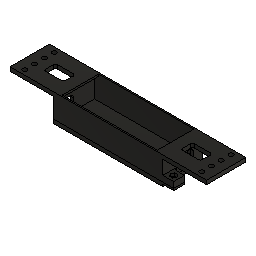
ports_usb_hub (Autodesk Fusion 360 design; units mm, degrees)
Autodesk Fusion 360 part; units mm, degrees
sketch "Sketch1" plane through (0, 0, 0) normal (0, 0, 1) x (1, 0, 0)
  line L0 (0, 0) -> (105, 0)
  line L1 (105, 0) -> (105, -36)
  line L2 (105, -36) -> (0, -36)
  line L3 (0, -36) -> (0, 0)
  line L4 (0, 0) -> (105, -36) construction
  line L5 (105, 0) -> (100, 0) construction
  line L6 (0, -36) -> (105, 0) construction
  line L7 (132.5, 2) -> (-27.5, 2)
  line L8 (-27.5, 2) -> (-27.5, -38)
  line L9 (-27.5, -38) -> (132.5, -38)
  line L10 (132.5, -38) -> (132.5, 2)
  line L11 (132.5, 2) -> (-27.5, -38) construction
  line L12 (-27.5, 2) -> (132.5, -38) construction
  line L13 (-27.5, 2) -> (-47.5, 2)
  line L14 (-47.5, 2) -> (-47.5, -38)
  line L15 (-47.5, -38) -> (-27.5, -38)
  line L16 (-27.5, -38) -> (-27.5, 2)
  line L17 (132.5, 2) -> (152.5, 2)
  line L18 (152.5, 2) -> (152.5, -38)
  line L19 (152.5, -38) -> (132.5, -38)
  line L20 (132.5, -38) -> (132.5, 2)
  line L21 (-37.5, 2) -> (-37.5, -38) construction
  line L22 (142.5, 2) -> (142.5, -38) construction
  line L23 (142.5, 2) -> (142.5, -3) construction
  line L24 (-37.5, 2) -> (-37.5, -3) construction
  circle A0 centre (142.5, -3) radius 2.2
  circle A1 centre (-37.5, -3) radius 2.2
  circle A2 centre (-37.5, -13) radius 2.2
  circle A3 centre (142.5, -13) radius 2.2
  circle A4 centre (-37.5, -23) radius 2.2
  circle A5 centre (142.5, -23) radius 2.2
  circle A6 centre (-37.5, -33) radius 2.2
  circle A7 centre (142.5, -33) radius 2.2
  line L25 (-3, 2) -> (108, 2)
  line L26 (108, 2) -> (108, -38)
  line L27 (108, -38) -> (-3, -38)
  line L28 (-3, -38) -> (-3, 2)
  line L29 (-3, 2) -> (108, -38) construction
  line L30 (108, 2) -> (-3, -38) construction
  point P0 (52.5, -18)
  point P1 (52.5, -18)
  dimension "d1" = 105
  dimension "d2" = 36
  dimension "d3" = 160
  dimension "d4" = 40
  dimension "d5" = 40
  dimension "d6" = 20
  dimension "d7" = 40
  dimension "d8" = 20
  dimension "d9" = 5
  dimension "d10" = 5
  dimension "d11" = 4.4
  dimension "d12" = 4.4
  dimension "d15" = 10
  dimension "d16" = -10
  dimension "d17" = 111
  dimension "d18" = 40
  constraint horizontal L0
  constraint vertical L1
  constraint horizontal L2
  constraint vertical L3
  constraint coincident L0.start L3.end
  constraint coincident L0 L5.end
  constraint perpendicular L7 L8
  constraint parallel L7 L9
  constraint parallel L8 L10
  constraint horizontal L7
  constraint coincident L11 P1
  constraint coincident L12 P1
  constraint midpoint L4 P1
  constraint horizontal L13
  constraint vertical L14
  constraint horizontal L15
  constraint vertical L16
  constraint horizontal L17
  constraint vertical L18
  constraint horizontal L19
  constraint vertical L20
  constraint midpoint L13 L21.start
  constraint midpoint L15 L21.end
  constraint midpoint L17 L22.start
  constraint midpoint L19 L22.end
  constraint perpendicular L17 L23
  constraint perpendicular L13 L24
  constraint coincident L23.end A0.centre
  constraint coincident L24.end A1.centre
  constraint perpendicular L25 L26
  constraint parallel L25 L27
  constraint parallel L26 L28
  constraint horizontal L25
  constraint coincident L29 P1
  constraint coincident L30 P1
  constraint coincident P1 P0
  measures "d1" distance of L0.start L0.end
  measures "d2" distance of L0.start L2.end
  measures "d3" distance of L8.end L9.end
  measures "d4" distance of L7.end L8.end
  measures "d5" distance of L7.end L8.end
  measures "d6" distance of L7.end L13.end
  measures "d7" distance of L7.start L9.end
  measures "d8" distance of L7.start L17.end
  measures "d9" distance of L22.start L23.end
  measures "d10" distance of L21.start L24.end
  measures "d11" diameter of A0
  measures "d12" diameter of A1
  measures "d17" distance of L26.end L27.end
  measures "d18" distance of L25.end L26.end
extrude "Extrude1" add sketch "Sketch1" along normal blind 4 makes body 1
extrude "Extrude2" add sketch "Sketch1" against normal blind 20 contours L7 L9 L25 L26 L27 L28 bodies 1
sketch "Sketch2" plane through (0, 0, -20) normal (0, 0, -1) x (1, 0, 0)
  line L0 (0, 36) -> (105, 36)
  line L1 (105, 36) -> (105, 0)
  line L2 (105, 0) -> (0, 0)
  line L3 (0, 0) -> (0, 36)
  line L4 (108, 38) -> (-3, 38)
  line L5 (-3, 38) -> (-3, -2)
  line L6 (-3, -2) -> (108, -2)
  line L7 (108, -2) -> (108, 38)
  line L8 (108, -2) -> (108, 7) construction
  line L9 (108, 7) -> (105, 7)
  line L10 (105, 7) -> (105, 15)
  line L11 (105, 15) -> (108, 15)
  line L12 (108, 15) -> (108, 7)
  line L13 (-3, 38) -> (-3, 29) construction
  line L14 (-3, 29) -> (0, 29)
  line L15 (0, 29) -> (0, 21)
  line L16 (0, 21) -> (-3, 21)
  line L17 (-3, 21) -> (-3, 29)
  dimension "d23" = 9
  dimension "d24" = 8
  dimension "d25" = 9
  dimension "d26" = 8
  constraint coincident L6.end L7.start
  constraint perpendicular L6 L8
  constraint horizontal L9
  constraint vertical L10
  constraint horizontal L11
  constraint vertical L12
  constraint coincident L4.end L5.start
  constraint perpendicular L4 L13
  constraint horizontal L14
  constraint vertical L15
  constraint horizontal L16
  constraint vertical L17
  measures "d23" distance of L6.end L8.end
  measures "d24" distance of L8.end L11.end
  measures "d25" distance of L4.end L13.end
  measures "d26" distance of L13.end L16.end
extrude "Extrude3" cut sketch "Sketch2" against normal blind 15 contours L3 L5 L14 L15 L16 L17 | L1 L7 L9 L10 L11 L12 bodies 1
fillet "Fillet1" radius 3 2 edges at (-1.5, -21, -5) (-1.5, -29, -5) on bodies 1
fillet "Fillet1" radius 3 2 edges at (106.5, -7, -5) (106.5, -15, -5) on bodies 1
sketch "Sketch3" plane through (0, 0, 4) normal (0, 0, 1) x (-1, 0, 0)
  circle A0 centre (-142.5, 33) radius 2.2
  circle A1 centre (37.5, 33) radius 2.2
  circle A2 centre (-142.5, 13) radius 2.2
  circle A3 centre (37.5, 23) radius 2.2
  circle A4 centre (-142.5, 23) radius 2.2
  circle A5 centre (37.5, 13) radius 2.2
  circle A6 centre (37.5, 3) radius 2.2
  circle A7 centre (-142.5, 3) radius 2.2
  line L0 (-105, 36) -> (0, 36)
  line L1 (0, 36) -> (0, 0)
  line L2 (0, 0) -> (-105, 0)
  line L3 (-105, 0) -> (-105, 36)
  line L4 (-152.5, -2) -> (47.5, -2)
  line L5 (47.5, -2) -> (47.5, 38)
  line L6 (47.5, 38) -> (-152.5, 38)
  line L7 (-152.5, 38) -> (-152.5, -2)
  line L8 (-52.5, 0) -> (-52.5, 36) construction
  line L9 (0, 0) -> (-3, 0)
  line L10 (-3, 0) -> (-3, 36)
  line L11 (-3, 36) -> (0, 36)
  line L12 (0, 36) -> (0, 0)
  line L13 (-102, 0) -> (-102, 36)
  dimension "d30" = 3
  constraint midpoint L2 L8.start
  constraint midpoint L0 L8.end
  constraint horizontal L9
  constraint vertical L10
  constraint horizontal L11
  constraint vertical L12
  constraint coincident L1.end L2.start
  constraint symmetric L8 L9.end L13.start
  constraint symmetric L8 L10.end L13.end
  measures "d30" distance of L1.end L9.end
extrude "Extrude4" add sketch "Sketch3" against normal blind 2 contours L0 L2 L3 L13 | L0 L1 L2 L9 L10 L11 L12 bodies 1
sketch "Sketch4" plane through (0, 0, -20) normal (0, 0, -1) x (1, 0, 0)
  line L0 (105, 7) -> (105, 0)
  line L1 (105, 0) -> (0, 0)
  line L2 (0, 0) -> (0, 21)
  line L3 (-3, 21) -> (-3, -2)
  line L4 (-3, -2) -> (108, -2)
  line L5 (108, -2) -> (108, 7)
  line L6 (0, 21) -> (-11, 21)
  line L7 (-11, 21) -> (-11, 10)
  line L8 (-11, 10) -> (0, 10)
  line L9 (0, 10) -> (0, 21)
  line L10 (0, 21) -> (-11, 10) construction
  circle A0 centre (-5.5, 15.5) radius 1.75
  line L11 (108, 7) -> (105, 7)
  line L12 (0, 21) -> (-3, 21)
  dimension "d33" = 11
  dimension "d34" = 11
  dimension "d35" = 3.5
  constraint horizontal L6
  constraint vertical L7
  constraint horizontal L8
  constraint vertical L9
  constraint coincident L2.end L6.start
  constraint midpoint L10 A0.centre
  measures "d33" distance of L2.end L6.end
  measures "d34" distance of L2.end L8.end
  measures "d35" diameter of A0
sketch "Sketch5" plane through (0, 0, -20) normal (0, 0, -1) x (1, 0, 0)
  line L0 (108, 7) -> (105, 7)
  line L1 (105, 7) -> (105, 0)
  line L2 (105, 0) -> (0, 0)
  line L3 (0, 0) -> (0, 21)
  line L4 (0, 21) -> (-3, 21)
  line L5 (-3, 21) -> (-3, -2)
  line L6 (-3, -2) -> (108, -2)
  line L7 (108, -2) -> (108, 7)
  line L8 (-3, -2) -> (-14, -2)
  line L9 (-14, -2) -> (-14, 9)
  line L10 (-14, 9) -> (-3, 9)
  line L11 (-3, 9) -> (-3, -2)
  circle A0 centre (-8.5, 3.5) radius 1.75
  dimension "d37" = 11
  dimension "d38" = 11
  dimension "d39" = 3.5
  constraint horizontal L8
  constraint vertical L9
  constraint horizontal L10
  constraint vertical L11
  constraint coincident L5.end L6.start
  measures "d37" distance of L5.end L10.end
  measures "d38" distance of L5.end L8.end
  measures "d39" diameter of A0
extrude "Extrude5" add sketch "Sketch5" against normal blind 20 separate body contours L5 L8 L9 L10 L11 makes body 2
sketch "Sketch6" plane through (0, 2, 0) normal (0, 1, 0) x (-1, 0, 0)
  line L0 (3, -20) -> (14, -20)
  line L1 (14, -20) -> (14, 0)
  line L2 (14, 0) -> (3, 0)
  line L3 (3, 0) -> (3, -20)
  line L4 (3, -20) -> (14, -20)
  line L5 (14, -20) -> (14, -17)
  line L6 (14, -17) -> (3, -17)
  line L7 (3, -17) -> (3, -20)
  line L8 (3, -17) -> (14, -17)
  line L9 (14, -17) -> (14, -14)
  line L10 (14, -14) -> (3, -14)
  line L11 (3, -14) -> (3, -17)
  dimension "d42" = 3
  dimension "d43" = 3
  constraint horizontal L4
  constraint vertical L5
  constraint horizontal L6
  constraint vertical L7
  constraint coincident L0.start L3.end
  constraint horizontal L8
  constraint vertical L9
  constraint horizontal L10
  constraint vertical L11
  measures "d42" distance of L0.start L6.end
  measures "d43" distance of L6.end L10.end
extrude "Extrude6" cut sketch "Sketch6" against normal blind 17.5 contours L1 L2 L3 L10 bodies 2
sketch "Sketch7" plane through (0, 0, -14) normal (0, 0, 1) x (-1, 0, 0)
  line L0 (14, 9) -> (3, 9)
  line L1 (3, 9) -> (3, -2)
  line L2 (3, -2) -> (14, -2)
  line L3 (14, -2) -> (14, 9)
  circle A0 centre (8.5, 3.5) radius 1.75
  line L4 (10.1166, 0.7) -> (11.7332, 3.5)
  line L5 (11.7332, 3.5) -> (10.1166, 6.3)
  line L6 (10.1166, 6.3) -> (6.8834, 6.3)
  line L7 (6.8834, 6.3) -> (5.2668, 3.5)
  line L8 (5.2668, 3.5) -> (6.8834, 0.7)
  line L9 (6.8834, 0.7) -> (10.1166, 0.7)
  point P0 (8.5, 3.5)
  dimension "d46" = 2.8
  constraint coincident P0 A0.centre
  measures "d46" distance of P0 L9
extrude "Extrude7" cut sketch "Sketch7" against normal blind 3 contours L4 L5 L6 L7 L8 L9 bodies 2
copy_body "CopyPasteBodies1" bodies 2 makes body 3
move_body "Move1" bodies 3 to x (1, 0, 0) y (0, 1, 0) z (0, 0, 1) at (122, -29, 0)
sketch "Sketch8" plane through (0, 0, -20) normal (0, 0, -1) x (1, 0, 0)
  circle A0 centre (-8.5, 3.5) radius 1.75
  line L0 (-3, 9) -> (-14, 9)
  line L1 (-14, 9) -> (-14, -2)
  line L2 (-14, -2) -> (-3, -2)
  line L3 (-3, -2) -> (-3, 9)
  line L4 (119, 27) -> (108, 27)
  line L5 (108, 27) -> (108, 38)
  line L6 (108, 38) -> (119, 38)
  line L7 (119, 38) -> (119, 27)
  line L8 (108, 38) -> (-3, 38)
  line L9 (-3, 38) -> (-3, -2)
  line L10 (-3, -2) -> (108, -2)
  line L11 (108, -2) -> (108, 38)
  circle A1 centre (-8.5, 3.5) radius 1.75
  circle A2 centre (113.5, 32.5) radius 1.75
  dimension "d49" = 3.5
  constraint horizontal L4
  constraint vertical L5
  constraint horizontal L6
  constraint vertical L7
  constraint horizontal L8
  constraint vertical L9
  constraint horizontal L10
  constraint vertical L11
  constraint coincident L2.end L3.start
  constraint concentric A0 A1
  measures "d49" diameter of A2
extrude "Extrude8" add sketch "Sketch8" along normal blind 2 separate body makes body 4
copy_body "Body->Comp1" bodies 1 removing the originals makes body 5 in component "Hub Mount"
copy_body "Body->Comp1'" bodies 5 removing the originals makes body 6 in component "Front"
copy_body "CutPasteBodies1" bodies 2 3 removing the originals makes body 7 makes body 8 in component "Front"
copy_body "Body->Comp2" bodies 4 removing the originals makes body 9 in component "Back plate"
sketch "Sketch9" plane through (0, 0, 4) normal (0, 0, 1) x (-1, 0, 0)
  circle A0 centre (-142.5, 33) radius 2.2
  circle A1 centre (37.5, 33) radius 2.2
  circle A2 centre (-142.5, 23) radius 2.2
  circle A3 centre (37.5, 23) radius 2.2
  circle A4 centre (-142.5, 13) radius 2.2
  circle A5 centre (37.5, 13) radius 2.2
  circle A6 centre (37.5, 3) radius 2.2
  circle A7 centre (-142.5, 3) radius 2.2
  line L0 (-102, 36) -> (-3, 36)
  line L1 (-3, 36) -> (-3, 0)
  line L2 (-3, 0) -> (-102, 0)
  line L3 (-102, 0) -> (-102, 36)
  line L4 (-152.5, -2) -> (47.5, -2)
  line L5 (47.5, -2) -> (47.5, 38)
  line L6 (47.5, 38) -> (-152.5, 38)
  line L7 (-152.5, 38) -> (-152.5, -2)
  line L8 (-52.5, -2) -> (-52.5, 38) construction
  line L9 (-152.5, 18) -> (47.5, 18) construction
  line L10 (47.5, 18) -> (27.5, 18) construction
  line L11 (27.5, 18) -> (27.5, -2) construction
  line L12 (27.5, 18) -> (27.5, 38) construction
  line L13 (7, -2) -> (7, 38) construction
  line L14 (7, 38) -> (27.5, -2) construction
  line L15 (25.25, 12) -> (9.25, 12)
  line L16 (7.25, 14) -> (7.25, 22)
  line L17 (9.25, 24) -> (25.25, 24)
  line L18 (27.25, 22) -> (27.25, 14)
  line L19 (27.25, 12) -> (7.25, 24) construction
  line L20 (7.25, 12) -> (27.25, 24) construction
  arc A8 (25.25, 12) -> (27.25, 14) centre (25.25, 14) ccw
  arc A9 (7.25, 14) -> (9.25, 12) centre (9.25, 14) ccw
  arc A10 (9.25, 24) -> (7.25, 22) centre (9.25, 22) ccw
  arc A11 (27.25, 22) -> (25.25, 24) centre (25.25, 22) ccw
  arc A12 (-114.25, 12) -> (-112.25, 14) centre (-114.25, 14) ccw
  line L21 (-112.25, 14) -> (-112.25, 22)
  arc A13 (-112.25, 22) -> (-114.25, 24) centre (-114.25, 22) ccw
  line L22 (-114.25, 24) -> (-130.25, 24)
  arc A14 (-130.25, 24) -> (-132.25, 22) centre (-130.25, 22) ccw
  line L23 (-132.25, 22) -> (-132.25, 14)
  arc A15 (-132.25, 14) -> (-130.25, 12) centre (-130.25, 14) ccw
  line L24 (-130.25, 12) -> (-114.25, 12)
  point P0 (17.25, 18)
  dimension "d52" = 20
  dimension "d53" = 20
  dimension "d54" = 12
  dimension "d55" = 2
  constraint midpoint L4 L8.start
  constraint midpoint L6 L8.end
  constraint midpoint L7 L9.start
  constraint midpoint L5 L9.end
  constraint perpendicular L5 L10
  constraint coincident L4 L11.end
  constraint perpendicular L4 L11
  constraint coincident L6 L12.end
  constraint perpendicular L6 L12
  constraint coincident L4 L13.start
  constraint coincident L6 L13.end
  constraint perpendicular L6 L13
  constraint perpendicular L15 L16
  constraint parallel L15 L17
  constraint parallel L16 L18
  constraint horizontal L15
  constraint coincident L19 P0
  constraint coincident L20 P0
  constraint midpoint L14 P0
  constraint coincident L19.start L18
  constraint coincident L19.start L15
  constraint tangent L18 A8
  constraint tangent L15 A8
  constraint coincident L20.start L16
  constraint coincident L20.start L15
  constraint tangent L16 A9
  constraint tangent L15 A9
  constraint equal A8 A9
  constraint coincident L19.end L17
  constraint coincident L19.end L16
  constraint tangent L17 A10
  constraint tangent L16 A10
  constraint equal A8 A10
  constraint coincident L20.end L17
  constraint coincident L20.end L18
  constraint tangent L17 A11
  constraint tangent L18 A11
  constraint equal A8 A11
  constraint symmetric L8 L18.end L23.end
  constraint symmetric L8 L15.start A15.end
  constraint symmetric L8 A8 A15
  constraint symmetric L8 L16.start A12.end
  constraint symmetric L8 L15.end A12.start
  constraint symmetric L8 A9 A12
  constraint symmetric L8 L17.start A13.end
  constraint symmetric L8 L16.end L21.end
  constraint symmetric L8 A10 A13
  constraint symmetric L8 L17.end L22.end
  constraint symmetric L8 L18.start A14.end
  constraint symmetric L8 A11 A14
  measures "d52" distance of L9.end L10.end
  measures "d53" distance of L19.end L20.end
  measures "d54" distance of L20.start L19.end
  measures "d55" radius of A8
extrude "Extrude1'" cut sketch "Sketch9" against normal blind 20 contours L15 L16 L17 L18 A8 A9 A10 A11 | A12 L21 A13 L22 A14 L23 A15 L24 bodies 6 in component "Front"
combine "Combine1" operation add target body 6 tool bodies 8 7 in component "Front"
fillet "Fillet1'" radius 3 1 edges at (-3, -9, -21) on bodies 9 in component "Back plate"
fillet "Fillet1''" radius 3 1 edges at (108, -27, -17) on bodies 6 in component "Front"
fillet "Fillet2" radius 3 1 edges at (108, -27, -21) on bodies 9 in component "Back plate"
fillet "Fillet2'" radius 3 1 edges at (-3, -9, -17) on bodies 6 in component "Front"
sketch "Sketch10" plane through (0, 0, -22) normal (0, 0, -1) x (1, 0, 0)
  circle A0 centre (113.5, 32.5) radius 1.75
  circle A1 centre (-8.5, 3.5) radius 1.75
  line L0 (119, 38) -> (-3, 38)
  line L1 (-3, 38) -> (-3, 12)
  arc A2 (-6, 9) -> (-3, 12) centre (-6, 12) ccw
  line L2 (-6, 9) -> (-14, 9)
  line L3 (-14, 9) -> (-14, -2)
  line L4 (-14, -2) -> (108, -2)
  line L5 (108, -2) -> (108, 24)
  arc A3 (111, 27) -> (108, 24) centre (111, 24) ccw
  line L6 (111, 27) -> (119, 27)
  line L7 (119, 27) -> (119, 38)
  line L8 (-3, 38) -> (108, 38) construction
  line L9 (108, 38) -> (108, -2) construction
  line L10 (108, -2) -> (-3, -2) construction
  line L11 (-3, -2) -> (-3, 38) construction
  line L12 (-3, 38) -> (108, 38)
  line L13 (108, 38) -> (108, 35)
  line L14 (108, 35) -> (-3, 35)
  line L15 (-3, 35) -> (-3, 38)
  line L16 (108, 16.5) -> (-3, 16.5)
  line L17 (-3, 16.5) -> (-3, 19.5)
  line L18 (-3, 19.5) -> (108, 19.5)
  line L19 (108, -2) -> (-3, -2)
  line L20 (-3, -2) -> (-3, 1)
  line L21 (-3, 1) -> (108, 1)
  line L22 (-3, 38) -> (0, 38)
  line L23 (0, 38) -> (0, -2)
  line L24 (0, -2) -> (-3, -2)
  line L25 (-3, -2) -> (-3, 38)
  line L26 (108, 38) -> (105, 38)
  line L27 (105, 38) -> (105, -2)
  line L28 (105, -2) -> (108, -2)
  line L29 (108, -2) -> (108, 38)
  line L30 (52.5, 19.5) -> (52.5, 16.5) construction
  line L31 (51, 38) -> (54, 38)
  line L32 (54, 38) -> (54, -2)
  line L33 (54, -2) -> (51, -2)
  line L34 (51, -2) -> (51, 38)
  line L35 (51, 38) -> (54, -2) construction
  line L36 (54, 38) -> (51, -2) construction
  point P0 (52.5, 18)
  dimension "d62" = 3
  dimension "d65" = 0
  dimension "d66" = -37
  dimension "d69" = 3
  constraint horizontal L8
  constraint vertical L9
  constraint horizontal L10
  constraint vertical L11
  constraint coincident L4.end L5.start
  constraint coincident L0.end L1.start
  constraint horizontal L12
  constraint vertical L13
  constraint horizontal L14
  constraint vertical L15
  constraint horizontal L22
  constraint vertical L23
  constraint horizontal L24
  constraint vertical L25
  constraint coincident L4 L23.end
  constraint horizontal L26
  constraint vertical L27
  constraint horizontal L28
  constraint vertical L29
  constraint midpoint L18 L30.start
  constraint midpoint L16 L30.end
  constraint perpendicular L31 L32
  constraint parallel L31 L33
  constraint parallel L32 L34
  constraint horizontal L31
  constraint coincident L12 L31.start
  constraint coincident L35 P0
  constraint coincident L36 P0
  constraint midpoint L30 P0
  measures "d62" distance of L0.end L14.end
  measures "d69" distance of L8.end L26.end
extrude "Extrude1''" add sketch "Sketch10" along normal blind 2 contours L0 L12 L13 L14 L26 L27 L29 | L0 L12 L14 L27 L32 | L5 L14 L18 L27 L29 | L0 L12 L14 L31 L32 L34 | L0 L12 L14 L23 L34 | L5 L16 L18 L27 L29 | L0 L1 L12 L14 L15 L22 L23 L25 | L5 L16 L21 L27 L29 | L1 L14 L18 L23 L25 | L4 L19 L21 L27 L32 | L4 L5 L19 L21 L27 L28 L29 | L1 L16 L17 L18 L23 L25 | L4 L19 L21 L32 L33 L34 | L1 L16 L21 L23 L25 | L4 L19 L21 L23 L34 | L4 L19 L20 L21 L23 L24 L25 bodies 9 in component "Back plate"
fillet "Fillet3" radius 3 4 edges at (0, -1, -23) (0, -35, -23) (105, -35, -23) (105, -1, -23) on bodies 9 in component "Back plate"
extrude "Extrude2'" add 1 faces at (102, -12, 2.6667) along direction (-1, 0, 0) blind 1 on bodies 6 bodies 6 in component "Front"
extrude "Extrude3'" add 1 faces at (3, -12, 2.6667) along direction (1, 0, 0) blind 1 on bodies 6 bodies 6 in component "Front"
sketch "Sketch11" plane through (0, 0, -22) normal (0, 0, -1) x (1, 0, 0)
  arc A0 (102, 1) -> (105, 4) centre (102, 4) ccw
  line L0 (105, 4) -> (105, 32)
  arc A1 (105, 32) -> (102, 35) centre (102, 32) ccw
  line L1 (102, 35) -> (3, 35)
  arc A2 (3, 35) -> (0, 32) centre (3, 32) ccw
  line L2 (0, 32) -> (0, 4)
  arc A3 (0, 4) -> (3, 1) centre (3, 4) ccw
  line L3 (3, 1) -> (102, 1)
  line L4 (3, 35) -> (102, 35) construction
  line L5 (102, 35) -> (102, 1) construction
  line L6 (102, 1) -> (3, 1) construction
  line L7 (3, 1) -> (3, 35) construction
  line L8 (102, 1) -> (3, 35) construction
  line L9 (3, 1) -> (102, 35) construction
  constraint horizontal L4
  constraint vertical L5
  constraint horizontal L6
  constraint vertical L7
  constraint coincident A0.start L3.end
  constraint coincident L1.end A2.start
  constraint coincident A3.end L3.start
extrude "Extrude4'" cut 1 faces at (36.3333, -36, -12.6667) along direction (0, -1, 0) blind 0.6 on bodies 6 bodies 6 in component "Front"
extrude "Extrude5'" cut 1 faces at (68.6667, 0, -12.6667) along direction (0, 1, 0) blind 0.6 on bodies 6 bodies 6 in component "Front"
extrude "Extrude6'" cut 1 faces at (105, -29.4, -8.6667) along direction (1, 0, 0) blind 0.2 on bodies 6 bodies 6 in component "Front"
extrude "Extrude7'" cut 1 faces at (0, -6.6, -8.6667) along direction (-1, 0, 0) blind 0.2 on bodies 6 bodies 6 in component "Front"
component "Hub Mount" placed x (1, 0, 0) y (0, 1, 0) z (0, 0, 1) at (0, 0, 0)
component "Front" placed x (1, 0, 0) y (0, 1, 0) z (0, 0, 1) at (0, 0, 0) in component "Hub Mount"
component "Back plate" placed x (1, 0, 0) y (0, 1, 0) z (0, 0, 1) at (0, 0, 0) in component "Hub Mount"
equation "d27 = -22 mm + 7 mm"
equation "d66 = -40.00 mm + 3 mm"
